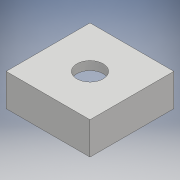
# Autodesk Inventor part: lupa_camera_mount
Saved by Autodesk Inventor 2018 (Build 220112000, 112)
## iProperties
Created: 2018-01-19
Part Number: lupa_camera_mount
Material: Generic
Document SubType Name: Modeling
Designer: matth
Density: 1 g/cm^3
Appearance: Default
Author: matth
Autodesk Inventor part; units mm, degrees
ref_plane "YZ Plane" through (0, 0, 0) normal (1, 0, 0) x (0, 1, 0)
ref_plane "XZ Plane" through (0, 0, 0) normal (0, 1, 0) x (-1, 0, 0)
ref_plane "XY Plane" through (0, 0, 0) normal (0, 0, 1) x (1, 0, 0)
sketch "Sketch1" plane through (0, 0, 0) normal (0, 0, 1) x (1, 0, 0)
  line L0 (-11.7234, 6.1825) -> (24.1766, 6.1825)
  line L1 (24.1766, 6.1825) -> (24.1766, -29.7175)
  line L2 (24.1766, -29.7175) -> (-11.7234, -29.7175)
  line L3 (-11.7234, -29.7175) -> (-11.7234, 6.1825)
  line L4 (-13.2234, 7.6825) -> (25.6766, 7.6825)
  line L5 (25.6766, 7.6825) -> (25.6766, -31.2175)
  line L6 (25.6766, -31.2175) -> (-13.2234, -31.2175)
  line L7 (-13.2234, -31.2175) -> (-13.2234, 7.6825)
  point P0 (0, 0)
  dimension "d0" = 35.9
  dimension "d1" = 35.9
  dimension "d2" = 38.9
  dimension "d3" = 38.9
  dimension "d4" = 1.5
  dimension "d5" = 1.5
  constraints: 16 end point, 4 parallel, 2 horizontal, 2 perpendicular
  measures "d0" distance of L1.end L2.end
  measures "d1" distance of L0.end L1.end
  measures "d2" distance of L5.end L6.end
  measures "d3" distance of L4.end L5.end
  measures "d4" distance between parallel lines of L4 L0
  measures "d5" distance between parallel lines of L7 L3
extrude "Extrusion1" add sketch "Sketch1" along normal blind 14
sketch "Sketch2" plane through (0, 0, 14) normal (0, 0, 1) x (1, 0, 0)
  line L0 (-13.2234, -31.2175) -> (-13.2234, 7.6825) projected
  line L1 (-13.2234, -31.2175) -> (25.6766, -31.2175) projected
  line L2 (-13.2234, 7.6825) -> (25.6766, 7.6825)
  line L3 (25.6766, 7.6825) -> (25.6766, -31.2175)
  line L4 (25.6766, -31.2175) -> (-13.2234, -31.2175)
  line L5 (-13.2234, -31.2175) -> (-13.2234, 7.6825)
  point P0 (0, 0)
  constraints: 8 end point, 2 parallel, 1 horizontal, 1 perpendicular
extrude "Extrusion2" add sketch "Sketch2" along normal blind 1
sketch "Sketch3" plane through (0, 0, 15) normal (0, 0, 1) x (1, 0, 0)
  circle A0 centre (6.2266, -11.7675) radius 6.1
  line L0 (-13.2234, 7.6825) -> (-13.2234, -31.2175) projected
  line L1 (-13.2234, -31.2175) -> (25.6766, -31.2175) projected
  point P0 (0, 0)
  dimension "d10" = 12.2
  dimension "d11" = 19.45
  dimension "d12" = 19.45
  dimension "d13" = 38.9
  constraints: 1 centre point
  measures "d10" diameter of A0
  measures "d11" distance from line of L0 A0.centre
  measures "d12" distance from line of L1 A0.centre
  measures "d13" distance of L0.start L0.end
extrude "Extrusion3" cut sketch "Sketch3" against normal blind 1
sketch "Sketch4" plane through (0, 0, 14) normal (0, 0, -1) x (-1, 0, 0)
  circle A0 centre (-6.2266, -11.7675) radius 6.1 projected
  circle A1 centre (-6.2266, -11.7675) radius 7.1
  point P0 (0, 0)
  dimension "d16" = 14.2
  constraints: 1 centre point, 1 coincident
  measures "d16" diameter of A1
extrude "Extrusion4" add sketch "Sketch4" along normal blind 3
fillet "Fillet1" radius 2 1 edges at (13.3266, -11.7675, 14)
sketch "Sketch5" plane through (0, 0, 14) normal (0, 0, -1) x (-1, 0, 0)
  line L0 (-24.1766, -29.7175) -> (11.7234, -29.7175) projected
  line L1 (11.7234, -29.7175) -> (9.7234, -29.7175)
  line L2 (9.7234, -29.7175) -> (11.7234, -27.7175)
  line L3 (11.7234, -29.7175) -> (11.7234, 6.1825) projected
  line L4 (11.7234, -27.7175) -> (11.7234, -29.7175)
  line L5 (11.7234, -29.7175) -> (11.7234, -27.7175)
  circle A0 centre (-6.2266, -11.7675) radius 6.1 projected
  line L6 (11.7234, 6.1825) -> (11.7234, 4.1825)
  line L7 (9.7234, 6.1825) -> (11.7234, 6.1825)
  line L8 (11.7234, 4.1825) -> (9.7234, 6.1825)
  line L9 (-24.1766, 6.1825) -> (-22.1766, 6.1825)
  line L10 (-24.1766, 4.1825) -> (-24.1766, 6.1825)
  line L11 (-22.1766, 6.1825) -> (-24.1766, 4.1825)
  line L12 (-24.1766, -29.7175) -> (-24.1766, -27.7175)
  line L13 (-22.1766, -29.7175) -> (-24.1766, -29.7175)
  line L14 (-24.1766, -27.7175) -> (-22.1766, -29.7175)
  point P0 (0, 0)
  dimension "d20" = 2
  dimension "d21" = 45
  dimension "d24" = 360
  constraints: 26 end point, 2 collinear, 2 point on line, 25 other
  measures "d20" distance of L0.end L1.end
  measures "d21" angle of L1 L2
extrude "Extrusion5" add sketch "Sketch5" along normal blind 12.5 contours L12 L14 L0 | L2 L3 L0 | L8 L7 L3 | L9 L11 L10
equation "\"d11\" = 0.5 * d13"
equation "\"d12\" = 0.5 * d13"
body "Solid1"
